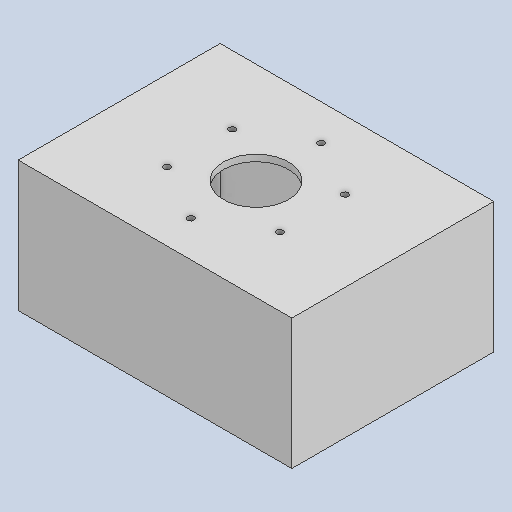
# Autodesk Inventor part: motor_holder
Saved by Autodesk Inventor 2025.3 (Build 293356030, 356C)
## iProperties
Created: 2025-08-30
Part Number: motor_holder
Material: 일반
Document SubType Name: Modeling
Designer: MSI
Density: 1 g/cm^3
Appearance: 기본값
Author: MSI
Autodesk Inventor part; units mm, degrees
ref_plane "YZ Plane" through (0, 0, 0) normal (1, 0, 0) x (0, 1, 0)
ref_plane "XZ Plane" through (0, 0, 0) normal (0, 1, 0) x (-1, 0, 0)
ref_plane "XY Plane" through (0, 0, 0) normal (0, 0, 1) x (1, 0, 0)
sketch "스케치1" plane through (0, 0, 0) normal (1, 0, 0) x (0, 1, 0)
  line L0 (50, 77.5) -> (-50, 77.5)
  line L1 (-50, 77.5) -> (-50, -77.5)
  line L2 (-50, -77.5) -> (50, -77.5)
  line L3 (50, -77.5) -> (50, 77.5)
  line L4 (50, 77.5) -> (-50, -77.5) construction
  line L5 (-50, 77.5) -> (50, -77.5) construction
  point P0 (0, 0)
  dimension "d0" = 100
  dimension "d1" = 155
  constraints: 12 end point, 2 midpoint, 2 parallel, 1 horizontal, 1 perpendicular
  measures "d0" distance of L2.end L1.end
  measures "d1" distance of L1.end L0.end
extrude "돌출1" add sketch "스케치1" against normal blind 105
shell "쉘1" thickness 5 removed faces 2 at (0, -16.6667, -25.8333) at (-35, -50, 25.8333)
sketch "스케치4" plane through (-100, 45, 77.5) normal (0, -1, 0) x (1, 0, 0)
  circle A0 centre (43, -47.5) radius 45
  line L0 (-5, 0) -> (-5, -155) projected
  line L1 (100, -155) -> (100, 0) projected
  point P0 (100, -77.5)
  point P1 (100, -77.5)
  dimension "d20" = 90
  dimension "d21" = 48
  dimension "d22" = 30
  constraints: 1 centre point, 1 midpoint
  measures "d20" diameter of A0
  measures "d21" distance from line of A0.centre L0
  measures "d22" vertical distance of point (100, -77.5) A0.centre
extrude "돌출3" cut sketch "스케치4" along normal blind 160
pattern_circular "원형 패턴2" count 2 over 360 about axis through (0, -10, 0) along (0, 1, 0)
sketch "스케치6" plane through (-105, 50, 77.5) normal (0, 1, 0) x (1, 0, 0)
  circle A0 centre (105, 77.5) radius 25
  dimension "d34" = 50
  constraints: 1 centre point, 1 coincident
  measures "d34" diameter of A0
extrude "돌출5" cut sketch "스케치6" against normal through all
sketch "스케치7" plane through (-105, 50, 77.5) normal (0, 1, 0) x (1, 0, 0)
  line L0 (105, 77.5) -> (105, 127.5) construction
  dimension "d37" = 50
  constraints: 2 end point, 1 vertical
  measures "d37" distance of L0.start L0.end
hole "구멍2" at (0, 50, -50) direction (0, -1, 0) diameter 5 end through all
pattern_circular "원형 패턴3" count 6 over 360 about axis through (0, 50, 0) along (0, -1, 0) of "구멍2"
